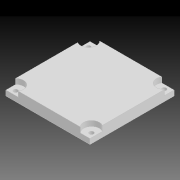
# Autodesk Inventor part: KB33-046-009 - Колпак лидара
Saved by Autodesk Inventor 2020 (Build 240168000, 168)
## iProperties
Created: 2021-08-10
Part Number: KB33-046-009 - Колпак лидара
Material: Типовые
Document SubType Name: Modeling
Designer: Петров Иван
Mass: 61.1507 g
Surface Area: 161.704 cm^2
Volume: 61.1507 cm^3
Density: 1 g/cm^3
Appearance: По умолчанию
Author: Петров Иван
Autodesk Inventor part; units mm, degrees
ref_plane "YZ Plane" through (0, 0, 0) normal (1, 0, 0) x (0, 1, 0)
ref_plane "XZ Plane" through (0, 0, 0) normal (0, 1, 0) x (-1, 0, 0)
ref_plane "XY Plane" through (0, 0, 0) normal (0, 0, 1) x (1, 0, 0)
sketch "Эскиз1" plane through (0, 0, 0) normal (0, 1, 0) x (-1, 0, 0)
  circle A0 centre (34.6317, 36.0644) radius 2
  circle A1 centre (-36.0644, 34.6317) radius 2
  circle A2 centre (-34.6317, -36.0644) radius 2
  circle A3 centre (36.0644, -34.6317) radius 2
  line L0 (-40, 40) -> (40, 40)
  line L1 (40, 40) -> (40, -40)
  line L2 (40, -40) -> (-40, -40)
  line L3 (-40, -40) -> (-40, 40)
  line L4 (-40, 40) -> (40, -40) construction
  line L5 (40, 40) -> (-40, -40) construction
  point P0 (0, 0)
  dimension "d0" = 4
  dimension "d1" = 50
  dimension "d4" = 360
  dimension "d6" = 80
  dimension "d7" = 80
  constraints: 12 end point, 4 centre point, 2 midpoint, 2 parallel, 1 horizontal, 1 perpendicular, 9 other
  measures "d0" diameter of A0
  measures "d1" distance of point (0, 0) A0.centre
  measures "d6" distance of L1.end L2.end
  measures "d7" distance of L0.end L1.end
extrude "Выдавливание1" add sketch "Эскиз1" along normal blind 10
sketch "Эскиз2" plane through (0, 10, 0) normal (0, 1, 0) x (1, 0, 0)
  circle A0 centre (-34.6317, -36.0644) radius 2 projected
  circle A1 centre (-34.6317, -36.0644) radius 7.5
  point P0 (0, 0)
  dimension "d10" = 15
  constraints: 1 centre point, 1 coincident
  measures "d10" diameter of A1
extrude "Выдавливание2" cut sketch "Эскиз2" against normal blind 5
pattern_circular "Круговой массив1" count 4 over 360 about axis through (0, -10, 0) along (0, 1, 0) of "Выдавливание2"
